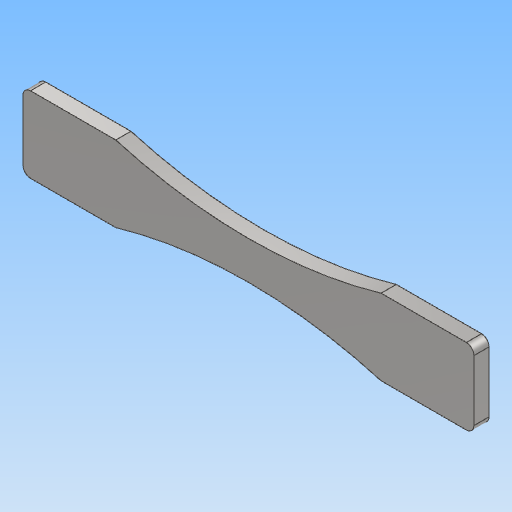
# Autodesk Inventor part: 0 零件
Saved by Autodesk Inventor 2020 (Build 240168000, 168)
## iProperties
Created: 2020-11-03
Part Number: 0 零件
Material: 不鏽鋼SUS-HL(砂紋)
Document SubType Name: Sheet Metal
Designer: p2013
Density: 8 g/cm^3
Appearance: 不鏽鋼 - 疏刷
Sheet Metal Rule: 預設 mm (_M)
Author: p2013
Autodesk Inventor part; units mm, degrees
ref_plane "YZ Plane" through (0, 0, 0) normal (1, 0, 0) x (0, 1, 0)
ref_plane "XZ Plane" through (0, 0, 0) normal (0, 1, 0) x (-1, 0, 0)
ref_plane "XY Plane" through (0, 0, 0) normal (0, 0, 1) x (1, 0, 0)
sketch "草圖1" plane through (0, 0, 0) normal (0, 0, 1) x (1, 0, 0)
  line L0 (0, 0) -> (-25.6572, 0) construction
  line L1 (0, 0) -> (0, 24.1407) construction
  line L2 (-28.75, -5) -> (28.75, -5)
  line L3 (29.75, -4) -> (29.75, 4)
  line L4 (28.75, 5) -> (-28.75, 5)
  line L5 (-29.75, 4) -> (-29.75, -4)
  line L6 (-29.75, -5) -> (29.75, 5) construction
  line L7 (29.75, -5) -> (-29.75, 5) construction
  arc A0 (28.75, -5) -> (29.75, -4) centre (28.75, -4) ccw
  arc A1 (-29.75, -4) -> (-28.75, -5) centre (-28.75, -4) ccw
  arc A2 (29.75, 4) -> (28.75, 5) centre (28.75, 4) ccw
  arc A3 (-28.75, 5) -> (-29.75, 4) centre (-28.75, 4) ccw
  arc A4 (-17.5, 5) -> (17.5, 5) centre (0, 65) ccw
  arc A5 (17.5, -5) -> (-17.5, -5) centre (0, -65) ccw
  point P0 (-17.5, -5)
  point P1 (17.5, -5)
  dimension "d0" = 59.5
  dimension "d1" = 10
  dimension "d4" = 1
  dimension "d5" = 1
  dimension "d8" = 5
  dimension "d9" = 35
  constraints: 16 end point, 12 point on circle, 10 point on line, 8 tangent, 6 centre point, 4 symmetric about line, 2 equal radius, 2 horizontal, 2 midpoint, 2 parallel, 1 perpendicular, 1 vertical, 1 other
  measures "d0" distance between parallel lines of L3 L5
  measures "d1" distance between parallel lines of L2 L4
  measures "d4" radius of A0
  measures "d5" radius of A2
  measures "d9" distance of A4.end A4.start
extrude "擠出1" add sketch "草圖1" along normal mid plane 2 contours A1 L5 A3 L4 A4 A2 L3 A0 L2 A5
equation "\"d4\" = d5"
equation "\"折彎半徑\" = 厚度"
equation "\"折彎離隙寬度\" = 厚度"
equation "\"折彎離隙深度\" = 0.5 * 厚度"
equation "\"轉角離隙大小\" = 4 * 厚度"
equation "\"最小剩餘\" = 2 * 厚度"
equation "\"轉移半徑\" = 折彎半徑"
equation "\"Jacobi半徑大小\" = 折彎半徑"
equation "\"間隙大小\" = 厚度"
equation "\"厚度\" = 2"
